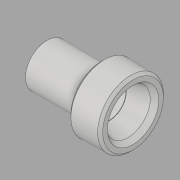
# Autodesk Inventor part: MS20819-2D
Saved by Autodesk Inventor 2019 (Build 230136000, 136)
## iProperties
Created: 2018-11-23
Part Number: MS20819-2D
Material: Aluminum 2014-T6
Document SubType Name: Modeling
Designer: erics
Mass: 0.30183 g
Surface Area: 2.77721 cm^2
Volume: 0.108211 cm^3
Density: 2.78927 g/cm^3
Appearance: Satin
Author: erics
Autodesk Inventor part; units mm, degrees
ref_plane "YZ Plane" through (0, 0, 0) normal (1, 0, 0) x (0, 1, 0)
ref_plane "XZ Plane" through (0, 0, 0) normal (0, 1, 0) x (-1, 0, 0)
ref_plane "XY Plane" through (0, 0, 0) normal (0, 0, 1) x (1, 0, 0)
sketch "Sketch1" plane through (0, 0, 0) normal (0, 0, 1) x (1, 0, 0)
  line L0 (0, 1.651) -> (6.3575, 1.651)
  line L1 (6.3978, 1.6576) -> (8.2197, 2.2672)
  line L2 (8.2197, 2.2672) -> (8.7376, 2.6035)
  line L3 (8.7376, 2.6035) -> (8.7376, 3.0815)
  line L4 (8.4836, 3.3399) -> (5.8166, 3.3865)
  line L5 (5.5626, 3.1369) -> (5.5626, 2.1844)
  line L6 (5.5626, 2.1844) -> (0, 2.1844)
  line L7 (0, 2.1844) -> (0, 1.651)
  line L8 (5.8166, 3.3865) -> (5.5626, 3.1369)
  line L9 (8.4836, 3.3399) -> (8.7376, 3.0815)
  arc A0 (6.3575, 1.651) -> (6.3978, 1.6576) centre (6.3575, 1.778) ccw
  line L10 (-6.035, 0) -> (36.2102, 0) projected
  point P0 (0, 0)
  point P1 (8.7376, 3.3355)
  point P2 (5.5626, 3.3909)
  dimension "d0" = 18.5
  dimension "d1" = 33
  dimension "d2" = 89
  dimension "d3" = 3.3909
  dimension "d4" = 2.1844
  dimension "d5" = 1.651
  dimension "d6" = 8.7376
  dimension "d7" = 2.6035
  dimension "d8" = 2.2672
  dimension "d9" = 3.175
  dimension "d10" = 0.254
  dimension "d11" = 0.254
  dimension "d12" = 0.254
  dimension "d13" = 0.254
  dimension "d14" = 0.127
  dimension "d16" = 0.0066
  constraints: 20 end point, 4 point on line, 3 perpendicular, 2 horizontal, 2 point on circle, 2 tangent, 1 centre point, 1 vertical alignment
  measures "d0" angle of L1 L0
  measures "d1" angle of L0 L2
  measures "d2" angle of L5 L4
  measures "d3" vertical distance of point (0, 0) point (5.563, 3.391)
  measures "d4" distance from line of point (0, 0) L6
  measures "d5" distance from line of point (0, 0) L0
  measures "d6" horizontal distance of point (0, 0) point (8.738, 3.335)
  measures "d7" vertical distance of point (0, 0) L2.end
  measures "d8" vertical distance of L1.end point (0, 0)
  measures "d9" distance between parallel lines of L3 L5
  measures "d10" distance of L4.end point (5.563, 3.391)
  measures "d11" distance of L5.start point (5.563, 3.391)
  measures "d12" distance of L4.start point (8.738, 3.335)
  measures "d13" distance of L3.end point (8.738, 3.335)
  measures "d14" radius of A0
  measures "d16" vertical distance of L1.start L0.end
revolve "Revolution1" add sketch "Sketch1" angle 360 about axis through (-10, 0, 0) along (1, 0, 0)
equation "\"d3\" = 0.5 * MS20819_G"
equation "\"d4\" = 0.5 * MS20819_C"
equation "\"d5\" = 0.5 * MS20819_B"
equation "\"d6\" = MS20819_M"
equation "\"d7\" = 0.5 * MS20819_F"
equation "\"d8\" = 0.5 * MS20819_N + d16"
equation "\"d9\" = MS20819_J"
equation "\"d11\" = d10"
equation "\"d12\" = d10"
equation "\"d13\" = d12"
equation "\"d14\" = MS20819_R"
equation "\"MS20819_B\" = 3.302"
equation "\"MS20819_C\" = 4.3688"
equation "\"MS20819_F\" = 5.207"
equation "\"MS20819_G\" = 6.7818"
equation "\"MS20819_J\" = 3.175"
equation "\"MS20819_M\" = 8.7376"
equation "\"MS20819_N\" = 4.5212"
equation "\"MS20819_R\" = 0.127"
equation "\"Tube_OD\" = 3.175"
body "Solid1"
